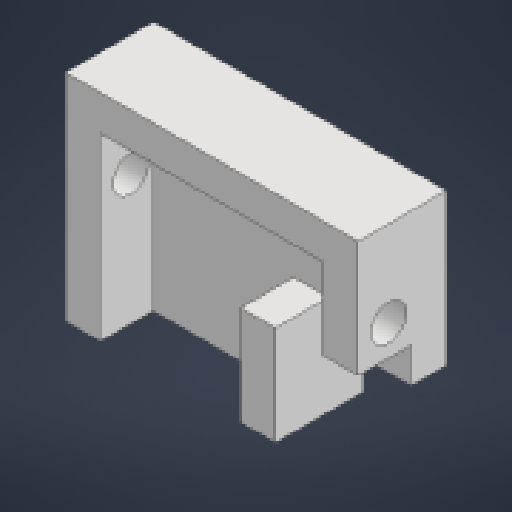
# Autodesk Inventor part: SS-5FL111-3T_Housing_01
Saved by Autodesk Inventor 2026.2 (Build 302298000, 298)
## iProperties
Created: 2026-02-23
Part Number: SS-5FL111-3T_Housing_01
Material: Generic
Document SubType Name: Modeling
Designer: vckot
Density: 1 g/cm^3
Appearance: Default
Author: vckot
Autodesk Inventor part; units mm, degrees
ref_plane "YZ Plane" through (0, 0, 0) normal (1, 0, 0) x (0, 1, 0)
ref_plane "XZ Plane" through (0, 0, 0) normal (0, 1, 0) x (-1, 0, 0)
ref_plane "XY Plane" through (0, 0, 0) normal (0, 0, 1) x (1, 0, 0)
sketch "Sketch1" plane through (0, 0, 0) normal (0, 0, 1) x (1, 0, 0)
  line L0 (4.1434, -12.66) -> (3.2904, -12.66)
  line L1 (-14.9, 12.8) -> (14.9, 12.8)
  line L2 (14.9, 12.8) -> (14.9, -12.8)
  line L3 (14.9, -12.8) -> (-14.9, -12.8)
  line L4 (-14.9, -12.8) -> (-14.9, 12.8)
  point P0 (0, 0)
  point P1 (0, 12.8)
  point P2 (-14.9, 0)
  dimension "d4" = 29.8
  dimension "d5" = 25.6
  constraints: 10 end point, 2 midpoint, 2 parallel, 1 horizontal, 1 horizontal alignment, 1 perpendicular, 1 vertical alignment
  measures "d4" distance of L1.start L1.end
  measures "d5" distance of L3.end L1.start
extrude "Extrusion1" add sketch "Sketch1" along normal blind 12.5
sketch "Sketch2" plane through (0, 0, 12.5) normal (0, 0, 1) x (1, 0, 0)
  line L0 (-14.9, -12.8) -> (14.9, -12.8) projected
  line L1 (-9.96, -12.8) -> (9.96, -12.8)
  line L2 (9.96, -12.8) -> (9.96, 7.8)
  line L3 (9.96, 7.8) -> (-9.96, 7.8)
  line L4 (-9.96, 7.8) -> (-9.96, -12.8)
  line L5 (14.9, 12.8) -> (-14.9, 12.8) projected
  point P0 (0, 0)
  point P1 (0, 7.8)
  dimension "d8" = 19.92
  dimension "d9" = 5
  constraints: 8 end point, 2 parallel, 1 horizontal, 1 midpoint, 1 perpendicular, 1 point on line, 1 vertical alignment
  measures "d8" distance of L2.end L3.end
  measures "d9" distance between parallel lines of L5 L3
extrude "Extrusion2" cut sketch "Sketch2" against normal blind 7.5
sketch "Sketch3" plane through (0, 0, 12.5) normal (0, 0, 1) x (1, 0, 0)
  line L0 (-0.14, 0.6) -> (-0.84, 1.3) projected
  line L1 (14.9, -12.8) -> (14.9, 12.8) projected
  line L2 (14.9, -3.7) -> (26.6432, -3.7)
  line L3 (26.6432, -3.7) -> (26.6432, 12.8)
  line L4 (26.6432, 12.8) -> (14.9, 12.8)
  line L5 (14.9, 12.8) -> (14.9, -3.7)
  line L6 (14.9, 12.8) -> (-14.9, 12.8) projected
  line L7 (-7.482, 1.9485) -> (17.86, 10.1145) projected
  line L8 (-7.482, 1.9485) -> (19.1432, 1.9485)
  line L9 (9.96, 7.8) -> (9.96, -12.8) projected
  line L10 (9.96, 1.3) -> (21.6432, 1.3)
  line L11 (21.6432, 1.3) -> (21.6432, 7.8)
  line L12 (21.6432, 7.8) -> (9.96, 7.8)
  line L13 (9.96, 7.8) -> (9.96, 1.3)
  line L14 (-9.96, 7.8) -> (9.96, 7.8) projected
  point P0 (0, 0)
  point P1 (15.8016, 1.3)
  point P2 (21.6432, 4.55)
  dimension "d12" = 5
  dimension "d13" = 7.5
  dimension "d14" = 5
  constraints: 18 end point, 4 parallel, 3 horizontal, 2 collinear, 2 midpoint, 2 perpendicular, 2 point on line, 1 equal length, 1 horizontal alignment
  measures "d12" distance from line of L2 L0.end
  measures "d13" distance from line of L3 L8.end
  measures "d14" distance from line of L3 point (21.643, 4.55)
extrude "Extrusion3" add sketch "Sketch3" against normal blind 12.5 contours L1 L10 L11 L12 L4 L3 L2 | L1 L12 L11 L10
sketch "Sketch4" plane through (0, 0, 12.5) normal (0, 0, 1) x (1, 0, 0)
  line L0 (21.6432, 7.8) -> (9.96, 7.8) projected
  line L1 (9.96, 7.8) -> (9.96, 1.3) projected
  line L2 (9.96, 1.3) -> (21.6432, 1.3) projected
  line L3 (21.6432, 1.3) -> (21.6432, 7.8) projected
  point P0 (0, 0)
extrude "Extrusion4" cut sketch "Sketch4" against normal blind 7.5
thicken "Thicken1" operation add thickness 5 both sides no extend neighbours no toward (0, 1, 0) faces at (12.7954, 12.8, 4.1667)
sketch "Sketch5" plane through (0, 0, 12.5) normal (0, 0, 1) x (1, 0, 0)
  line L0 (-9.96, 7.8) -> (21.6432, 7.8) projected
  line L1 (-9.96, 7.8) -> (21.6432, 7.8)
  line L2 (21.6432, 7.8) -> (21.6432, 12.8)
  line L3 (21.6432, 12.8) -> (-9.96, 12.8)
  line L4 (-9.96, 12.8) -> (-9.96, 7.8)
  line L5 (21.6432, 7.8) -> (21.6432, 1.3) projected
  point P0 (0, 0)
  dimension "d21" = 5
  constraints: 8 end point, 2 parallel, 1 collinear, 1 horizontal, 1 perpendicular
  measures "d21" distance of L2.end L1.end
extrude "Extrusion5" cut sketch "Sketch5" against normal blind 7.5
sketch "Sketch6" plane through (-14.9, -12.8, 0) normal (-1, 0, 0) x (0, 0, 1)
  circle A0 centre (8.2, 18.4735) radius 2.525
  line L0 (10, 14.7485) -> (6.4, 14.7485) projected
  line L1 (6.6, 15.3) -> (9.8, 15.3)
  point P0 (0, 12.8)
  point P1 (8.2, 14.7485)
  point P2 (8.2, 15.9485)
  dimension "d24" = 5.05
  dimension "d25" = 1.2
  constraints: 3 vertical alignment, 2 end point, 1 horizontal, 1 midpoint, 4 other
  measures "d25" distance from line of L0 point (8.2, 15.948)
extrude "Extrusion6" cut sketch "Sketch6" against normal through all
sketch "Sketch7" plane through (0, 0, 12.5) normal (0, 0, 1) x (1, 0, 0)
  line L0 (14.9, -3.7) -> (26.6432, -3.7) projected
  line L1 (26.6432, -3.7) -> (26.6432, 17.8) projected
  line L2 (14.9, -3.7) -> (26.6432, -3.7)
  line L3 (26.6432, -3.7) -> (26.6432, 1.3)
  line L4 (26.6432, 1.3) -> (14.9, 1.3)
  line L5 (14.9, 1.3) -> (14.9, -3.7)
  point P0 (0, 0)
  dimension "d28" = 5
  constraints: 8 end point, 2 parallel, 1 horizontal, 1 perpendicular, 1 point on line
  measures "d28" distance of L3.end L2.end
extrude "Extrusion7" cut sketch "Sketch7" against normal through all
body "Solid1"
